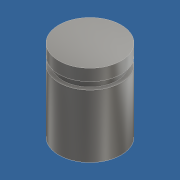
# Autodesk Inventor part: AxeJambe
Saved by Autodesk Inventor 2018 (Build 220112000, 112)
## iProperties
Created: 2022-04-05
Part Number: AxeJambe
Material: Stainless Steel
Document SubType Name: Modeling
Designer: Nathann
Density: 8 g/cm^3
Appearance: Semi-Polished
Mass: 3.89105 g
Surface Area: 3.91191 cm^2
Volume: 0.486381 cm^3
Author: Nathann
Autodesk Inventor part; units mm, degrees
ref_plane "YZ Plane" through (0, 0, 0) normal (1, 0, 0) x (0, 1, 0)
ref_plane "XZ Plane" through (0, 0, 0) normal (0, 1, 0) x (-1, 0, 0)
ref_plane "XY Plane" through (0, 0, 0) normal (0, 0, 1) x (1, 0, 0)
sketch "Sketch1" plane through (0, 0, 0) normal (0, 0, 1) x (1, 0, 0)
  circle A0 centre (0, 0) radius 4
  dimension "d0" = 8
  constraints: 1 centre point, 1 coincident
  measures "d0" diameter of A0
extrude "Extrusion1" add sketch "Sketch1" along normal blind 10.5
sketch "Sketch2" plane through (0, 0, 0) normal (1, 0, 0) x (0, 1, 0)
  line L0 (4.5, 9) -> (3.5, 9)
  line L1 (3.5, 9) -> (3.5, 8.06)
  line L2 (3.5, 8.06) -> (4.5, 8.06)
  line L3 (4.5, 8.06) -> (4.5, 9)
  line L4 (4, 0) -> (4, 10.5) projected
  line L5 (4, 10.5) -> (-4, 10.5) projected
  line L6 (0, -2.2) -> (0, 13.2) projected
  line L7 (2.4774, 8) -> (9.7598, 8) projected
  point P0 (0, 0)
  dimension "d3" = 0.5
  dimension "d4" = 1
  dimension "d5" = 0.94
  dimension "d6" = 1.5
  constraints: 8 end point, 2 parallel, 1 horizontal, 1 perpendicular
  measures "d3" distance between parallel lines of L4 L1
  measures "d4" distance of L0.start L0.end
  measures "d5" distance of L2.end L0.start
  measures "d6" distance between parallel lines of L5 L0
revolve "Revolution1" cut sketch "Sketch2" angle 360 about axis through (0, 0, -10) along (0, 0, 1)
equation "\"d4\" = 2 * d3"
body "Solid1"
